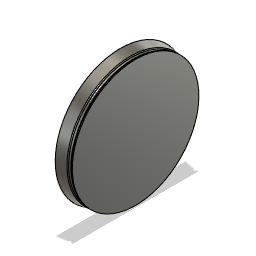
briefkasten_deckel (Autodesk Fusion 360 design; units mm, degrees)
Autodesk Fusion 360 part; units mm, degrees
note: some values were not read from the file. Set by a fixed rule: which sketch regions a step uses.
sketch "Skizze1" plane through (0, 0, 0) normal (0, 0, 1) x (1, 0, 0)
  line L0 (0, 0) -> (0, 50)
  line L1 (-12, 51.4988) -> (-12, 49.4043)
  line L2 (-12, 49.4043) -> (-1.2, 47.5)
  line L3 (-1.2, 47.5) -> (-1.2, 0)
  line L4 (-1.2, 0) -> (0, 0)
  line L5 (0, 50) -> (-1.5, 50)
  circle A0 centre (-2.5, 50) radius 1
  line L6 (-12, 51.4988) -> (-3.5, 50)
  dimension "d1" = 1.2
  dimension "d7" = 50
  dimension "d19" = 2
  dimension "d21" = 2.5
  dimension "d22" = 1.5
  dimension "d23" = 12
  dimension "d24" = 100
  constraint coincident L0.start L4.end
  constraint vertical L0
  constraint parallel L0 L3
  constraint perpendicular L0 L4
  constraint perpendicular L0 L5
  constraint coincident L5.end A0
  constraint coincident L5 A0.centre
  constraint coincident A0 L6.end
  constraint coincident L5 L6.end
  constraint coincident L1.start L6.start
  constraint parallel L2 L6
  measures "d1" distance of L3.end L0.start
  measures "d7" distance of L0.start L0.end
  measures "d19" diameter of A0
  measures "d21" distance of L2.end L5
  measures "d22" distance of L0.end L5.end
  measures "d23" distance of L0 L1
  measures "d24" angle of L3 L6
revolve "Drehen1" add sketch "Skizze1" angle 360 about axis through (-1.2, 0, 0) along (1, 0, 0) contours L0 L1 L2 L3 L4 L5 A0 L6
fillet "Abrundung1" radius 3 1 edges at (-1.2, -17.1767, 44.2855)
fillet "Abrundung2" radius 1 2 edges at (-3.5, -18.0808, 46.6164) (-1.5, -18.0808, 46.6164)
equation "d21 = d19 / 2 + 1.5 mm"
